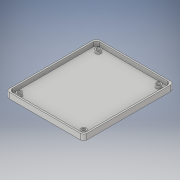
# Autodesk Inventor part: Buttom Part
Saved by Autodesk Inventor 2018.3 (Build 223284000, 284)
## iProperties
Created: 2019-10-06
Part Number: Buttom Part
Material: Generic
Document SubType Name: Modeling
Designer: Jamal Bouajjaj
Density: 1 g/cm^3
Appearance: Default
Author: Jamal Bouajjaj
Autodesk Inventor part; units mm, degrees
ref_plane "YZ Plane" through (0, 0, 0) normal (1, 0, 0) x (0, 1, 0)
ref_plane "XZ Plane" through (0, 0, 0) normal (0, 1, 0) x (-1, 0, 0)
ref_plane "XY Plane" through (0, 0, 0) normal (0, 0, 1) x (1, 0, 0)
sketch "Sketch1" plane through (0, 0, 0) normal (0, 1, 0) x (-1, 0, 0)
  line L0 (-2.54, -2.54) -> (-71.12, -2.54) construction
  line L1 (-71.12, -2.54) -> (-71.12, -83.185) construction
  line L2 (-71.12, -83.185) -> (-2.54, -83.185) construction
  line L3 (-2.54, -83.185) -> (-2.54, -2.54) construction
  circle A0 centre (-6.35, -6.35) radius 1.6
  circle A1 centre (-8.255, -79.375) radius 1.6
  circle A2 centre (-67.31, -6.35) radius 1.6
  circle A3 centre (-65.405, -79.375) radius 1.6
  line L4 (-8.255, -79.375) -> (-65.405, -79.375) construction
  line L5 (-6.35, -6.35) -> (-67.31, -6.35) construction
  line L6 (-6.35, -6.35) -> (-8.255, -79.375) construction
  line L7 (-67.31, -6.35) -> (-65.405, -79.375) construction
  line L8 (0, -85.725) -> (-73.66, -85.725)
  line L9 (-73.66, -85.725) -> (-73.66, 0)
  line L10 (-73.66, 0) -> (0, 0)
  line L11 (0, 0) -> (0, -85.725)
  line L12 (-2.54, -83.185) -> (0, -85.725) construction
  line L13 (-71.12, -83.185) -> (-73.66, -85.725) construction
  line L14 (-73.66, 0) -> (-71.12, -2.54) construction
  line L15 (0, 0) -> (-2.54, -2.54) construction
  line L16 (-1.5, -1.5) -> (-72.16, -1.5)
  line L17 (-72.16, -1.5) -> (-72.16, -84.225)
  line L18 (-72.16, -84.225) -> (-1.5, -84.225)
  line L19 (-1.5, -84.225) -> (-1.5, -1.5)
  circle A4 centre (-6.35, -6.35) radius 2.5
  circle A5 centre (-8.255, -79.375) radius 2.5
  circle A6 centre (-65.405, -79.375) radius 2.5
  circle A7 centre (-67.31, -6.35) radius 2.5
  dimension "d0" = 3.2
  dimension "d1" = 57.15
  dimension "d2" = 60.96
  dimension "d3" = 73.025
  dimension "d4" = 68.58
  dimension "d5" = 80.645
  dimension "d6" = 2.54
  dimension "d7" = 2.54
  dimension "d8" = 1.5
  dimension "d9" = 5
  dimension "d16" = 3.81
  dimension "d17" = 3.81
  dimension "d18" = 3.81
  constraints: 40 end point, 8 centre point, 6 equal radius, 6 parallel, 5 coincident, 5 horizontal, 4 equal length, 3 perpendicular, 3 point on line
  measures "d0" diameter of A1
  measures "d1" distance of L4.start L4.end
  measures "d2" distance of L5.start L5.end
  measures "d3" distance between parallel lines of L5 L4
  measures "d4" distance of L0.start L0.end
  measures "d5" distance of L2.end L0.start
  measures "d6" horizontal distance of L9.end L0.end
  measures "d7" horizontal distance of L9.end L0.end
  measures "d8" distance between parallel lines of L10 L16
  measures "d9" diameter of A5
  measures "d16" distance from line of L5.start L0
  measures "d17" distance from line of L2 L4.start
  measures "d18" distance from line of L3 A4.centre
extrude "Extrusion1" add sketch "Sketch1" against normal blind 1.27 contours L8 L9 L10 L11 | L19 L18 L17 L16
extrude "Extrusion2" add sketch "Sketch1" along normal blind 2.54
extrude "Extrusion3" add sketch "Sketch1" along normal blind 1.6 from surface at 2.54 contours L8 L9 L10 L11
fillet "Fillet1" radius 3.175 8 edges at (0, 1.435, 0) (1.5, 2.07, -1.5) (1.5, 2.07, -84.225) (0, 1.435, -85.725) (72.16, 2.07, -84.225) (73.66, 1.435, -85.725) (72.16, 2.07, -1.5) (73.66, 1.435, 0)
body "Solid1"
